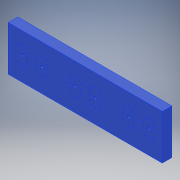
# Autodesk Inventor part: Gehaeuse_IN12_Fassung
Saved by Autodesk Inventor 2019 (Build 230136000, 136)
## iProperties
Created: 2019-10-07
Part Number: Gehaeuse_IN12_Fassung
Material: Generisch
Document SubType Name: Modeling
Designer: grubi
Density: 1 g/cm^3
Appearance: Vorgabe
Author: grubi
Autodesk Inventor part; units mm, degrees
ref_plane "YZ Plane" through (0, 0, 0) normal (1, 0, 0) x (0, 1, 0)
ref_plane "XZ Plane" through (0, 0, 0) normal (0, 1, 0) x (-1, 0, 0)
ref_plane "XY Plane" through (0, 0, 0) normal (0, 0, 1) x (1, 0, 0)
sketch "Skizze1" plane through (0, 0, 0) normal (0, 0, 1) x (1, 0, 0)
  spline S0 degree 3 poles (-66.4365, 60.4568) (-65.8605, 59.5154) (-65.2905, 58.8685) (-64.3775, 57.9498) (-63.6818, 57.3426) (-61.9226, 56.3485) (-61.068, 56.0155) (-59.0889, 55.5216) (-58.1394, 55.4718) (-57.6712, 55.4581) knots 0 0 0 0 0.331084 0.331084 0.698981 0.698981 1.004245 1.004245 1.384179 1.384179 1.384179 1.384179 projected
  line L0 (-57.6712, 55.4581) -> (-56.2137, 55.4552) projected
  spline S1 degree 3 poles (-56.2137, 55.4552) (-55.6042, 55.4706) (-54.6957, 55.5362) (-52.7979, 56.0044) (-51.9528, 56.3319) (-50.3662, 57.2202) (-49.6505, 57.7658) (-48.3993, 59.0179) (-47.8793, 59.6887) (-47.4285, 60.4187) knots 0 0 0 0 0.182919 0.182919 0.342589 0.342589 0.502166 0.502166 0.65206 0.65206 0.65206 0.65206 projected
  arc A0 (-47.4285, 60.4187) -> (-46.7276, 62.8786) centre (-51.4276, 62.888) ccw projected
  line L1 (-46.7276, 62.8786) -> (-46.6966, 78.3939) projected
  arc A1 (-46.6966, 78.3939) -> (-47.3876, 80.8565) centre (-51.3966, 78.4033) ccw projected
  spline S2 degree 3 poles (-47.3876, 80.8565) (-47.9637, 81.7979) (-48.5337, 82.4448) (-49.4467, 83.3635) (-50.1424, 83.9707) (-51.9015, 84.9648) (-52.7562, 85.2978) (-54.7353, 85.7917) (-55.6848, 85.8415) (-56.1529, 85.8552) knots 0 0 0 0 0.331084 0.331084 0.698981 0.698981 1.004245 1.004245 1.384179 1.384179 1.384179 1.384179 projected
  line L2 (-56.1529, 85.8552) -> (-57.6105, 85.8581) projected
  spline S3 degree 3 poles (-57.6105, 85.8581) (-58.22, 85.8427) (-59.1285, 85.7771) (-61.0263, 85.3089) (-61.8713, 84.9814) (-63.458, 84.0931) (-64.1737, 83.5475) (-65.4248, 82.2954) (-65.9449, 81.6246) (-66.3957, 80.8945) knots 0 0 0 0 0.182919 0.182919 0.342589 0.342589 0.502166 0.502166 0.65206 0.65206 0.65206 0.65206 projected
  arc A2 (-66.3957, 80.8945) -> (-67.0966, 78.4347) centre (-62.3966, 78.4253) ccw projected
  line L3 (-67.0966, 78.4347) -> (-67.1276, 62.9194) projected
  arc A3 (-67.1276, 62.9194) -> (-66.4365, 60.4568) centre (-62.4276, 62.91) ccw projected
  circle A4 centre (-60.9281, 62.6647) radius 0.5 projected
  circle A5 centre (-56.9301, 61.6567) radius 0.5 projected
  circle A6 centre (-52.9281, 62.6487) radius 0.5 projected
  circle A7 centre (-51.1711, 66.1452) radius 0.5 projected
  circle A8 centre (-51.1621, 70.6451) radius 0.5 projected
  circle A9 centre (-62.6711, 66.1682) radius 0.5 projected
  circle A10 centre (-62.6621, 70.6681) radius 0.5 projected
  circle A11 centre (-51.1531, 75.1451) radius 0.5 projected
  circle A12 centre (-52.8961, 78.6486) radius 0.5 projected
  circle A13 centre (-56.8941, 79.6566) radius 0.5 projected
  circle A14 centre (-62.6531, 75.1681) radius 0.5 projected
  circle A15 centre (-60.8961, 78.6646) radius 0.5 projected
  circle A16 centre (-56.9121, 70.6566) radius 1.45 projected
  spline S4 degree 3 poles (-45.6066, 60.4151) (-45.0305, 59.4738) (-44.4605, 58.8269) (-43.5475, 57.9082) (-42.8518, 57.3009) (-41.0927, 56.3068) (-40.2381, 55.9738) (-38.2589, 55.48) (-37.3094, 55.4301) (-36.8413, 55.4165) knots 0 0 0 0 0.331084 0.331084 0.698981 0.698981 1.004245 1.004245 1.384179 1.384179 1.384179 1.384179 projected
  line L4 (-36.8413, 55.4165) -> (-35.3838, 55.4136) projected
  spline S5 degree 3 poles (-35.3838, 55.4136) (-34.7742, 55.4289) (-33.8657, 55.4945) (-31.968, 55.9627) (-31.1229, 56.2903) (-29.5362, 57.1785) (-28.8206, 57.7241) (-27.5694, 58.9762) (-27.0493, 59.6471) (-26.5986, 60.3771) knots 0 0 0 0 0.182919 0.182919 0.342589 0.342589 0.502166 0.502166 0.65206 0.65206 0.65206 0.65206 projected
  arc A17 (-26.5986, 60.3771) -> (-25.8977, 62.8369) centre (-30.5977, 62.8463) ccw projected
  line L5 (-25.8977, 62.8369) -> (-25.8666, 78.3522) projected
  arc A18 (-25.8666, 78.3522) -> (-26.5577, 80.8149) centre (-30.5666, 78.3616) ccw projected
  spline S6 degree 3 poles (-26.5577, 80.8149) (-27.1337, 81.7562) (-27.7038, 82.4031) (-28.6167, 83.3218) (-29.3125, 83.929) (-31.0716, 84.9231) (-31.9262, 85.2561) (-33.9053, 85.75) (-34.8549, 85.7998) (-35.323, 85.8135) knots 0 0 0 0 0.331084 0.331084 0.698981 0.698981 1.004245 1.004245 1.384179 1.384179 1.384179 1.384179 projected
  line L6 (-35.323, 85.8135) -> (-36.7805, 85.8164) projected
  spline S7 degree 3 poles (-36.7805, 85.8164) (-37.39, 85.8011) (-38.2986, 85.7355) (-40.1963, 85.2672) (-41.0414, 84.9397) (-42.628, 84.0514) (-43.3437, 83.5058) (-44.5949, 82.2537) (-45.115, 81.5829) (-45.5657, 80.8529) knots 0 0 0 0 0.182919 0.182919 0.342589 0.342589 0.502166 0.502166 0.65206 0.65206 0.65206 0.65206 projected
  arc A19 (-45.5657, 80.8529) -> (-46.2666, 78.393) centre (-41.5666, 78.3836) ccw projected
  line L7 (-46.2666, 78.393) -> (-46.2976, 62.8777) projected
  arc A20 (-46.2976, 62.8777) -> (-45.6066, 60.4151) centre (-41.5976, 62.8683) ccw projected
  circle A21 centre (-40.0981, 62.623) radius 0.5 projected
  circle A22 centre (-36.1001, 61.615) radius 0.5 projected
  circle A23 centre (-32.0981, 62.607) radius 0.5 projected
  circle A24 centre (-30.3411, 66.1035) radius 0.5 projected
  circle A25 centre (-30.3321, 70.6035) radius 0.5 projected
  circle A26 centre (-41.8411, 66.1265) radius 0.5 projected
  circle A27 centre (-41.8321, 70.6265) radius 0.5 projected
  circle A28 centre (-30.3231, 75.1035) radius 0.5 projected
  circle A29 centre (-32.0661, 78.607) radius 0.5 projected
  circle A30 centre (-36.0641, 79.615) radius 0.5 projected
  circle A31 centre (-41.8231, 75.1265) radius 0.5 projected
  circle A32 centre (-40.0661, 78.623) radius 0.5 projected
  circle A33 centre (-36.0821, 70.615) radius 1.45 projected
  spline S8 degree 3 poles (-11.4366, 60.3468) (-10.8606, 59.4054) (-10.2906, 58.7585) (-9.3776, 57.8398) (-8.6819, 57.2326) (-6.9228, 56.2385) (-6.0681, 55.9055) (-4.089, 55.4116) (-3.1395, 55.3618) (-2.6714, 55.3481) knots 0 0 0 0 0.331084 0.331084 0.698981 0.698981 1.004245 1.004245 1.384179 1.384179 1.384179 1.384179 projected
  line L8 (-2.6714, 55.3481) -> (-1.2138, 55.3452) projected
  spline S9 degree 3 poles (-1.2138, 55.3452) (-0.6043, 55.3606) (0.3042, 55.4262) (2.202, 55.8944) (3.0471, 56.2219) (4.6337, 57.1102) (5.3494, 57.6558) (6.6006, 58.9079) (7.1206, 59.5787) (7.5714, 60.3088) knots 0 0 0 0 0.182919 0.182919 0.342589 0.342589 0.502166 0.502166 0.65206 0.65206 0.65206 0.65206 projected
  arc A34 (7.5714, 60.3088) -> (8.2723, 62.7686) centre (3.5723, 62.778) ccw projected
  line L9 (8.2723, 62.7686) -> (8.3033, 78.2839) projected
  arc A35 (8.3033, 78.2839) -> (7.6122, 80.7465) centre (3.6033, 78.2933) ccw projected
  spline S10 degree 3 poles (7.6122, 80.7465) (7.0362, 81.6879) (6.4662, 82.3348) (5.5532, 83.2535) (4.8575, 83.8607) (3.0984, 84.8548) (2.2437, 85.1878) (0.2646, 85.6817) (-0.6849, 85.7315) (-1.153, 85.7452) knots 0 0 0 0 0.331084 0.331084 0.698981 0.698981 1.004245 1.004245 1.384179 1.384179 1.384179 1.384179 projected
  line L10 (-1.153, 85.7452) -> (-2.6106, 85.7481) projected
  spline S11 degree 3 poles (-2.6106, 85.7481) (-3.2201, 85.7327) (-4.1286, 85.6671) (-6.0264, 85.1989) (-6.8715, 84.8714) (-8.4581, 83.9831) (-9.1738, 83.4375) (-10.425, 82.1854) (-10.945, 81.5146) (-11.3958, 80.7846) knots 0 0 0 0 0.182919 0.182919 0.342589 0.342589 0.502166 0.502166 0.65206 0.65206 0.65206 0.65206 projected
  arc A36 (-11.3958, 80.7846) -> (-12.0967, 78.3247) centre (-7.3967, 78.3153) ccw projected
  line L11 (-12.0967, 78.3247) -> (-12.1277, 62.8094) projected
  arc A37 (-12.1277, 62.8094) -> (-11.4366, 60.3468) centre (-7.4277, 62.8) ccw projected
  circle A38 centre (-5.9282, 62.5547) radius 0.5 projected
  circle A39 centre (-1.9302, 61.5467) radius 0.5 projected
  circle A40 centre (2.0718, 62.5387) radius 0.5 projected
  circle A41 centre (3.8288, 66.0352) radius 0.5 projected
  circle A42 centre (3.8378, 70.5352) radius 0.5 projected
  circle A43 centre (-7.6712, 66.0582) radius 0.5 projected
  circle A44 centre (-7.6622, 70.5582) radius 0.5 projected
  circle A45 centre (3.8468, 75.0351) radius 0.5 projected
  circle A46 centre (2.1038, 78.5386) radius 0.5 projected
  circle A47 centre (-1.8942, 79.5466) radius 0.5 projected
  circle A48 centre (-7.6532, 75.0581) radius 0.5 projected
  circle A49 centre (-5.8962, 78.5546) radius 0.5 projected
  circle A50 centre (-1.9122, 70.5467) radius 1.45 projected
  spline S12 degree 3 poles (9.3933, 60.3051) (9.9694, 59.3638) (10.5394, 58.7169) (11.4524, 57.7982) (12.1481, 57.1909) (13.9072, 56.1969) (14.7618, 55.8639) (16.7409, 55.37) (17.6905, 55.3202) (18.1586, 55.3065) knots 0 0 0 0 0.331084 0.331084 0.698981 0.698981 1.004245 1.004245 1.384179 1.384179 1.384179 1.384179 projected
  line L12 (18.1586, 55.3065) -> (19.6161, 55.3036) projected
  spline S13 degree 3 poles (19.6161, 55.3036) (20.2257, 55.3189) (21.1342, 55.3845) (23.0319, 55.8528) (23.877, 56.1803) (25.4636, 57.0685) (26.1793, 57.6142) (27.4305, 58.8662) (27.9506, 59.5371) (28.4013, 60.2671) knots 0 0 0 0 0.182919 0.182919 0.342589 0.342589 0.502166 0.502166 0.65206 0.65206 0.65206 0.65206 projected
  arc A51 (28.4013, 60.2671) -> (29.1022, 62.727) centre (24.4022, 62.7364) ccw projected
  line L13 (29.1022, 62.727) -> (29.1332, 78.2423) projected
  arc A52 (29.1332, 78.2423) -> (28.4422, 80.7049) centre (24.4333, 78.2517) ccw projected
  spline S14 degree 3 poles (28.4422, 80.7049) (27.8662, 81.6462) (27.2961, 82.2931) (26.3832, 83.2118) (25.6874, 83.8191) (23.9283, 84.8131) (23.0737, 85.1461) (21.0946, 85.64) (20.145, 85.6898) (19.6769, 85.7035) knots 0 0 0 0 0.331084 0.331084 0.698981 0.698981 1.004245 1.004245 1.384179 1.384179 1.384179 1.384179 projected
  line L14 (19.6769, 85.7035) -> (18.2194, 85.7064) projected
  spline S15 degree 3 poles (18.2194, 85.7064) (17.6099, 85.6911) (16.7013, 85.6255) (14.8036, 85.1573) (13.9585, 84.8297) (12.3719, 83.9415) (11.6562, 83.3958) (10.405, 82.1438) (9.8849, 81.4729) (9.4342, 80.7429) knots 0 0 0 0 0.182919 0.182919 0.342589 0.342589 0.502166 0.502166 0.65206 0.65206 0.65206 0.65206 projected
  arc A53 (9.4342, 80.7429) -> (8.7333, 78.2831) centre (13.4333, 78.2737) ccw projected
  line L15 (8.7333, 78.2831) -> (8.7023, 62.7677) projected
  arc A54 (8.7023, 62.7677) -> (9.3933, 60.3051) centre (13.4023, 62.7583) ccw projected
  circle A55 centre (14.9018, 62.513) radius 0.5 projected
  circle A56 centre (18.8998, 61.505) radius 0.5 projected
  circle A57 centre (22.9017, 62.497) radius 0.5 projected
  circle A58 centre (24.6587, 65.9935) radius 0.5 projected
  circle A59 centre (24.6677, 70.4935) radius 0.5 projected
  circle A60 centre (13.1588, 66.0165) radius 0.5 projected
  circle A61 centre (13.1678, 70.5165) radius 0.5 projected
  circle A62 centre (24.6767, 74.9935) radius 0.5 projected
  circle A63 centre (22.9337, 78.497) radius 0.5 projected
  circle A64 centre (18.9358, 79.505) radius 0.5 projected
  circle A65 centre (13.1768, 75.0165) radius 0.5 projected
  circle A66 centre (14.9338, 78.513) radius 0.5 projected
  circle A67 centre (18.9178, 70.505) radius 1.45 projected
  spline S16 degree 3 poles (43.5632, 60.2368) (44.1393, 59.2954) (44.7093, 58.6485) (45.6223, 57.7298) (46.318, 57.1226) (48.0771, 56.1285) (48.9318, 55.7955) (50.9109, 55.3016) (51.8604, 55.2518) (52.3285, 55.2382) knots 0 0 0 0 0.331084 0.331084 0.698981 0.698981 1.004245 1.004245 1.384179 1.384179 1.384179 1.384179 projected
  line L16 (52.3285, 55.2382) -> (53.786, 55.2352) projected
  spline S17 degree 3 poles (53.786, 55.2352) (54.3956, 55.2506) (55.3041, 55.3162) (57.2019, 55.7844) (58.0469, 56.1119) (59.6336, 57.0002) (60.3493, 57.5458) (61.6004, 58.7979) (62.1205, 59.4688) (62.5713, 60.1988) knots 0 0 0 0 0.182919 0.182919 0.342589 0.342589 0.502166 0.502166 0.65206 0.65206 0.65206 0.65206 projected
  arc A68 (62.5713, 60.1988) -> (63.2722, 62.6586) centre (58.5722, 62.668) ccw projected
  line L17 (63.2722, 62.6586) -> (63.3032, 78.1739) projected
  arc A69 (63.3032, 78.1739) -> (62.6121, 80.6366) centre (58.6032, 78.1833) ccw projected
  spline S18 degree 3 poles (62.6121, 80.6366) (62.0361, 81.5779) (61.4661, 82.2248) (60.5531, 83.1435) (59.8573, 83.7507) (58.0982, 84.7448) (57.2436, 85.0778) (55.2645, 85.5717) (54.3149, 85.6215) (53.8468, 85.6352) knots 0 0 0 0 0.331084 0.331084 0.698981 0.698981 1.004245 1.004245 1.384179 1.384179 1.384179 1.384179 projected
  line L18 (53.8468, 85.6352) -> (52.3893, 85.6381) projected
  spline S19 degree 3 poles (52.3893, 85.6381) (51.7798, 85.6227) (50.8713, 85.5571) (48.9735, 85.0889) (48.1284, 84.7614) (46.5418, 83.8731) (45.8261, 83.3275) (44.5749, 82.0754) (44.0549, 81.4046) (43.6041, 80.6746) knots 0 0 0 0 0.182919 0.182919 0.342589 0.342589 0.502166 0.502166 0.65206 0.65206 0.65206 0.65206 projected
  arc A70 (43.6041, 80.6746) -> (42.9032, 78.2147) centre (47.6032, 78.2053) ccw projected
  line L19 (42.9032, 78.2147) -> (42.8722, 62.6994) projected
  arc A71 (42.8722, 62.6994) -> (43.5632, 60.2368) centre (47.5722, 62.69) ccw projected
  circle A72 centre (49.0717, 62.4447) radius 0.5 projected
  circle A73 centre (53.0697, 61.4367) radius 0.5 projected
  circle A74 centre (57.0717, 62.4287) radius 0.5 projected
  circle A75 centre (58.8287, 65.9252) radius 0.5 projected
  circle A76 centre (58.8377, 70.4252) radius 0.5 projected
  circle A77 centre (47.3287, 65.9482) radius 0.5 projected
  circle A78 centre (47.3377, 70.4482) radius 0.5 projected
  circle A79 centre (58.8467, 74.9252) radius 0.5 projected
  circle A80 centre (57.1037, 78.4287) radius 0.5 projected
  circle A81 centre (53.1057, 79.4367) radius 0.5 projected
  circle A82 centre (47.3467, 74.9482) radius 0.5 projected
  circle A83 centre (49.1037, 78.4447) radius 0.5 projected
  circle A84 centre (53.0877, 70.4367) radius 1.45 projected
  spline S20 degree 3 poles (64.3932, 60.1951) (64.9692, 59.2538) (65.5393, 58.6069) (66.4522, 57.6882) (67.148, 57.081) (68.9071, 56.0869) (69.7617, 55.7539) (71.7408, 55.26) (72.6904, 55.2102) (73.1585, 55.1965) knots 0 0 0 0 0.331084 0.331084 0.698981 0.698981 1.004245 1.004245 1.384179 1.384179 1.384179 1.384179 projected
  line L20 (73.1585, 55.1965) -> (74.616, 55.1936) projected
  spline S21 degree 3 poles (74.616, 55.1936) (75.2255, 55.2089) (76.1341, 55.2745) (78.0318, 55.7428) (78.8769, 56.0703) (80.4635, 56.9586) (81.1792, 57.5042) (82.4304, 58.7563) (82.9505, 59.4271) (83.4012, 60.1571) knots 0 0 0 0 0.182919 0.182919 0.342589 0.342589 0.502166 0.502166 0.65206 0.65206 0.65206 0.65206 projected
  arc A85 (83.4012, 60.1571) -> (84.1021, 62.617) centre (79.4021, 62.6264) ccw projected
  line L21 (84.1021, 62.617) -> (84.1331, 78.1323) projected
  arc A86 (84.1331, 78.1323) -> (83.4421, 80.5949) centre (79.4331, 78.1417) ccw projected
  spline S22 degree 3 poles (83.4421, 80.5949) (82.866, 81.5362) (82.296, 82.1831) (81.383, 83.1018) (80.6873, 83.7091) (78.9282, 84.7032) (78.0736, 85.0362) (76.0945, 85.53) (75.1449, 85.5799) (74.6768, 85.5935) knots 0 0 0 0 0.331084 0.331084 0.698981 0.698981 1.004245 1.004245 1.384179 1.384179 1.384179 1.384179 projected
  line L22 (74.6768, 85.5935) -> (73.2193, 85.5964) projected
  spline S23 degree 3 poles (73.2193, 85.5964) (72.6097, 85.5811) (71.7012, 85.5155) (69.8035, 85.0473) (68.9584, 84.7197) (67.3718, 83.8315) (66.6561, 83.2859) (65.4049, 82.0338) (64.8848, 81.3629) (64.4341, 80.6329) knots 0 0 0 0 0.182919 0.182919 0.342589 0.342589 0.502166 0.502166 0.65206 0.65206 0.65206 0.65206 projected
  arc A87 (64.4341, 80.6329) -> (63.7332, 78.1731) centre (68.4332, 78.1637) ccw projected
  line L23 (63.7332, 78.1731) -> (63.7022, 62.6578) projected
  arc A88 (63.7022, 62.6578) -> (64.3932, 60.1951) centre (68.4021, 62.6484) ccw projected
  circle A89 centre (69.9017, 62.403) radius 0.5 projected
  circle A90 centre (73.8996, 61.395) radius 0.5 projected
  circle A91 centre (77.9016, 62.387) radius 0.5 projected
  circle A92 centre (79.6586, 65.8835) radius 0.5 projected
  circle A93 centre (79.6676, 70.3835) radius 0.5 projected
  circle A94 centre (68.1587, 65.9065) radius 0.5 projected
  circle A95 centre (68.1677, 70.4065) radius 0.5 projected
  circle A96 centre (79.6766, 74.8835) radius 0.5 projected
  circle A97 centre (77.9336, 78.387) radius 0.5 projected
  circle A98 centre (73.9356, 79.395) radius 0.5 projected
  circle A99 centre (68.1767, 74.9065) radius 0.5 projected
  circle A100 centre (69.9337, 78.403) radius 0.5 projected
  circle A101 centre (73.9176, 70.395) radius 1.45 projected
  line L24 (8.5956, 101.4703) -> (8.3793, 37.8364)
  line L25 (87.7471, 92.8448) -> (-70.7709, 92.8448)
  line L26 (-70.7709, 92.8448) -> (-70.7709, 46.8448)
  line L27 (-70.7709, 46.8448) -> (87.7471, 46.8448)
  line L28 (87.7471, 46.8448) -> (87.7471, 92.8448)
  line L29 (87.7471, 92.8448) -> (-70.7709, 46.8448) construction
  line L30 (-70.7709, 92.8448) -> (87.7471, 46.8448) construction
  line L31 (-12.3093, 46.9974) -> (32.6286, 46.9075) projected
  line L32 (32.8464, 92.2972) -> (-12.2185, 92.3873) projected
  point P0 (0, 0)
  point P1 (8.4881, 69.8448)
  dimension "d0" = 46
  constraints: 14 end point, 2 midpoint, 2 parallel, 1 horizontal, 1 perpendicular, 1 point on line, 3 other
  measures "d0" distance of L27.end L25.start
extrude "Extrusion2" add sketch "Skizze1" along normal blind 4 contours A3 L3 A2 S3 L2 S2 A1 L1 A0 S1 L0 S0 | A20 L7 A19 S7 L6 S6 A18 L5 A17 S5 L4 S4 | A37 L11 A36 S11 L10 S10 A35 L9 A34 S9 L8 S8 | A54 L15 A53 S15 L14 S14 A52 L13 A51 S13 L12 S12 | A71 L19 A70 S19 L18 S18 A69 L17 A68 S17 L16 S16 | A88 L23 A87 S23 L22 S22 A86 L21 A85 S21 L20 S20 | L25 L28 L27 L24 | L24 L27 L26 L25
sketch "Skizze2" plane through (0, 0, 4) normal (0, 0, 1) x (1, 0, 0)
  spline S0 degree 3 poles (73.1538, 54.8965) (72.9276, 54.903) (72.6988, 54.9155) (72.4727, 54.9339) (70.685, 55.0793) (68.9331, 55.6222) (67.4319, 56.598) (66.2444, 57.37) (65.2425, 58.3865) (64.4481, 59.5565) (64.3411, 59.7141) (64.2375, 59.8748) (64.1373, 60.0385) knots 0 0 0 0 0.000679 0.000679 0.000679 0.006047 0.006047 0.006047 0.010293 0.010293 0.010293 0.010865 0.010865 0.010865 0.010865 projected
  line L0 (74.6195, 54.8936) -> (73.1538, 54.8965) projected
  spline S1 degree 3 poles (83.6565, 59.9995) (83.5977, 59.9044) (83.5358, 59.807) (83.4115, 59.6178) (83.2216, 59.3372) (83.0208, 59.0664) (82.6043, 58.5384) (82.3068, 58.2044) (81.6695, 57.5748) (81.3297, 57.2792) (80.6038, 56.7301) (80.2221, 56.4801) (79.4273, 56.0341) (79.017, 55.8396) (78.1797, 55.5075) (77.7515, 55.3692) (76.877, 55.1452) (76.4287, 55.0593) (75.5277, 54.9393) (75.0747, 54.9049) (74.6195, 54.8936) knots 0 0 0 0 0.000335 0.000335 0.000671 0.001342 0.001342 0.002684 0.002684 0.004025 0.004025 0.005367 0.005367 0.006709 0.006709 0.008051 0.008051 0.009392 0.009392 0.010734 0.010734 0.010734 0.010734 projected
  arc A0 (83.6565, 59.9995) -> (84.4021, 62.6164) centre (79.4021, 62.6264) ccw projected
  line L1 (84.4331, 78.1317) -> (84.4021, 62.6164) projected
  arc A1 (84.4331, 78.1317) -> (83.698, 80.7515) centre (79.4331, 78.1417) ccw projected
  spline S2 degree 3 poles (74.6814, 85.8935) (74.9077, 85.887) (75.1365, 85.8746) (75.3626, 85.8562) (77.1503, 85.7107) (78.9022, 85.1678) (80.4033, 84.192) (81.5909, 83.42) (82.5928, 82.4036) (83.3872, 81.2336) (83.4942, 81.076) (83.5978, 80.9152) (83.698, 80.7515) knots 0 0 0 0 0.000679 0.000679 0.000679 0.006047 0.006047 0.006047 0.010293 0.010293 0.010293 0.010865 0.010865 0.010865 0.010865 projected
  line L2 (73.2158, 85.8964) -> (74.6814, 85.8935) projected
  spline S3 degree 3 poles (64.1788, 80.7905) (64.2376, 80.8857) (64.2995, 80.983) (64.4237, 81.1722) (64.6137, 81.4529) (64.8145, 81.7236) (65.231, 82.2516) (65.5285, 82.5856) (66.1658, 83.2152) (66.5056, 83.5108) (67.2315, 84.06) (67.6132, 84.3099) (68.4079, 84.7559) (68.8183, 84.9505) (69.6556, 85.2826) (70.0838, 85.4208) (70.9583, 85.6449) (71.4066, 85.7308) (72.3076, 85.8507) (72.7606, 85.8851) (73.2158, 85.8964) knots 0 0 0 0 0.000335 0.000335 0.000671 0.001342 0.001342 0.002684 0.002684 0.004025 0.004025 0.005367 0.005367 0.006709 0.006709 0.008051 0.008051 0.009392 0.009392 0.010734 0.010734 0.010734 0.010734 projected
  arc A2 (64.1788, 80.7905) -> (63.4332, 78.1737) centre (68.4332, 78.1637) ccw projected
  arc A3 (63.4022, 62.6584) -> (64.1373, 60.0385) centre (68.4021, 62.6484) ccw projected
  line L3 (63.4022, 62.6584) -> (63.4332, 78.1737) projected
  point P0 (0, 0)
extrude "Extrusion3" cut sketch "Skizze2" against normal through all
sketch "Skizze3" plane through (0, 0, 4) normal (0, 0, 1) x (1, 0, 0)
  spline S0 degree 3 poles (53.8515, 85.9352) (54.0777, 85.9287) (54.3065, 85.9162) (54.5327, 85.8978) (56.3203, 85.7524) (58.0723, 85.2095) (59.5734, 84.2336) (60.7609, 83.4616) (61.7628, 82.4452) (62.5572, 81.2752) (62.6642, 81.1176) (62.7678, 80.9569) (62.868, 80.7931) knots 0 0 0 0 0.000679 0.000679 0.000679 0.006047 0.006047 0.006047 0.010293 0.010293 0.010293 0.010865 0.010865 0.010865 0.010865 projected
  line L0 (52.3859, 85.9381) -> (53.8515, 85.9352) projected
  spline S1 degree 3 poles (43.3489, 80.8322) (43.4076, 80.9273) (43.4695, 81.0247) (43.5938, 81.2139) (43.7837, 81.4945) (43.9846, 81.7653) (44.4011, 82.2933) (44.6985, 82.6273) (45.3358, 83.2569) (45.6756, 83.5525) (46.4016, 84.1016) (46.7832, 84.3516) (47.578, 84.7976) (47.9883, 84.9921) (48.8256, 85.3242) (49.2538, 85.4625) (50.1283, 85.6865) (50.5766, 85.7724) (51.4776, 85.8924) (51.9306, 85.9268) (52.3859, 85.9381) knots 0 0 0 0 0.000335 0.000335 0.000671 0.001342 0.001342 0.002684 0.002684 0.004025 0.004025 0.005367 0.005367 0.006709 0.006709 0.008051 0.008051 0.009392 0.009392 0.010734 0.010734 0.010734 0.010734 projected
  arc A0 (43.3489, 80.8322) -> (42.6032, 78.2153) centre (47.6032, 78.2053) ccw projected
  line L1 (42.5722, 62.7) -> (42.6032, 78.2153) projected
  arc A1 (42.5722, 62.7) -> (43.3074, 60.0802) centre (47.5722, 62.69) ccw projected
  spline S2 degree 3 poles (52.3239, 54.9382) (52.0976, 54.9447) (51.8689, 54.9571) (51.6427, 54.9755) (49.8551, 55.121) (48.1031, 55.6639) (46.602, 56.6397) (45.4144, 57.4117) (44.4125, 58.4281) (43.6181, 59.5981) (43.5111, 59.7557) (43.4076, 59.9164) (43.3074, 60.0802) knots 0 0 0 0 0.000679 0.000679 0.000679 0.006047 0.006047 0.006047 0.010293 0.010293 0.010293 0.010865 0.010865 0.010865 0.010865 projected
  line L2 (53.7895, 54.9352) -> (52.3239, 54.9382) projected
  spline S3 degree 3 poles (62.8265, 60.0412) (62.7678, 59.946) (62.7058, 59.8487) (62.5816, 59.6594) (62.3916, 59.3788) (62.1908, 59.1081) (61.7743, 58.5801) (61.4769, 58.246) (60.8396, 57.6164) (60.4997, 57.3209) (59.7738, 56.7717) (59.3921, 56.5218) (58.5974, 56.0758) (58.1871, 55.8812) (57.3497, 55.5491) (56.9215, 55.4108) (56.0471, 55.1868) (55.5987, 55.1009) (54.6978, 54.981) (54.2448, 54.9465) (53.7895, 54.9352) knots 0 0 0 0 0.000335 0.000335 0.000671 0.001342 0.001342 0.002684 0.002684 0.004025 0.004025 0.005367 0.005367 0.006709 0.006709 0.008051 0.008051 0.009392 0.009392 0.010734 0.010734 0.010734 0.010734 projected
  arc A2 (62.8265, 60.0412) -> (63.5722, 62.658) centre (58.5722, 62.668) ccw projected
  line L3 (63.6032, 78.1733) -> (63.5722, 62.658) projected
  arc A3 (63.6032, 78.1733) -> (62.868, 80.7931) centre (58.6032, 78.1833) ccw projected
  point P0 (0, 0)
extrude "Extrusion4" cut sketch "Skizze3" against normal through all
sketch "Skizze4" plane through (0, 0, 4) normal (0, 0, 1) x (1, 0, 0)
  spline S0 degree 3 poles (19.6816, 86.0035) (19.9078, 85.997) (20.1366, 85.9846) (20.3627, 85.9662) (22.1504, 85.8207) (23.9023, 85.2778) (25.4035, 84.302) (26.591, 83.53) (27.5929, 82.5136) (28.3873, 81.3436) (28.4943, 81.1859) (28.5979, 81.0252) (28.6981, 80.8615) knots 0 0 0 0 0.000679 0.000679 0.000679 0.006047 0.006047 0.006047 0.010293 0.010293 0.010293 0.010865 0.010865 0.010865 0.010865 projected
  spline S1 degree 3 poles (18.2159, 86.0064) (18.21, 86.0063) (18.2038, 86.0061) (18.1971, 86.006) (18.1703, 86.0053) (18.1437, 86.0045) (18.1172, 86.0036) (18.0632, 86.0019) (18.0099, 85.9998) (17.9571, 85.9975) (17.8473, 85.9926) (17.7402, 85.9865) (17.6353, 85.9792) (17.4098, 85.9636) (17.1947, 85.9427) (16.985, 85.9171) (16.5342, 85.8619) (16.1111, 85.7864) (15.6701, 85.6799) (15.2325, 85.5742) (14.7906, 85.4387) (14.3636, 85.2757) (13.9278, 85.1095) (13.4975, 84.911) (13.0876, 84.6856) (12.2663, 84.2341) (11.5215, 83.6759) (10.8506, 83.0137) (10.2077, 82.3792) (9.6538, 81.6696) (9.1789, 80.9005) knots 0 0 0 0 0.000018 0.000018 0.000018 0.000088 0.000088 0.000088 0.000233 0.000233 0.000233 0.000534 0.000534 0.000534 0.001182 0.001182 0.001182 0.002574 0.002574 0.002574 0.003955 0.003955 0.003955 0.005365 0.005365 0.005365 0.008189 0.008189 0.008189 0.010895 0.010895 0.010895 0.010895 projected
  line L0 (18.2159, 86.0064) -> (19.6816, 86.0035) projected
  arc A0 (29.4332, 78.2417) -> (28.6981, 80.8615) centre (24.4333, 78.2517) ccw projected
  line L1 (29.4332, 78.2417) -> (29.4022, 62.7264) projected
  arc A1 (28.6566, 60.1095) -> (29.4022, 62.7264) centre (24.4022, 62.7364) ccw projected
  spline S2 degree 3 poles (28.6566, 60.1095) (28.5978, 60.0143) (28.5359, 59.917) (28.4117, 59.7278) (28.2217, 59.4472) (28.0209, 59.1764) (27.6044, 58.6484) (27.3069, 58.3144) (26.6696, 57.6848) (26.3298, 57.3892) (25.6039, 56.8401) (25.2222, 56.5901) (24.4275, 56.1441) (24.0171, 55.9496) (23.1798, 55.6174) (22.7516, 55.4792) (21.8771, 55.2552) (21.4288, 55.1692) (20.5278, 55.0493) (20.0748, 55.0149) (19.6196, 55.0036) knots 0 0 0 0 0.000335 0.000335 0.000671 0.001342 0.001342 0.002684 0.002684 0.004025 0.004025 0.005367 0.005367 0.006709 0.006709 0.008051 0.008051 0.009392 0.009392 0.010734 0.010734 0.010734 0.010734 projected
  line L2 (19.6196, 55.0036) -> (18.154, 55.0065) projected
  spline S3 degree 3 poles (18.154, 55.0065) (17.9277, 55.013) (17.6989, 55.0254) (17.4728, 55.0438) (15.6851, 55.1893) (13.9332, 55.7322) (12.4321, 56.708) (11.2445, 57.48) (10.2426, 58.4964) (9.4482, 59.6664) (9.3412, 59.8241) (9.2376, 59.9848) (9.1374, 60.1485) knots 0 0 0 0 0.000679 0.000679 0.000679 0.006047 0.006047 0.006047 0.010293 0.010293 0.010293 0.010865 0.010865 0.010865 0.010865 projected
  arc A2 (8.4023, 62.7683) -> (9.1374, 60.1485) centre (13.4023, 62.7583) ccw projected
  line L3 (8.4023, 62.7683) -> (8.4333, 78.2837) projected
  arc A3 (9.1789, 80.9005) -> (8.4333, 78.2837) centre (13.4333, 78.2737) ccw projected
  spline S4 degree 3 poles (-1.1484, 86.0452) (-0.9221, 86.0386) (-0.6934, 86.0262) (-0.4672, 86.0078) (1.3204, 85.8623) (3.0724, 85.3195) (4.5735, 84.3436) (5.761, 83.5716) (6.7629, 82.5552) (7.5573, 81.3852) (7.6644, 81.2276) (7.7679, 81.0669) (7.8681, 80.9031) knots 0 0 0 0 0.000679 0.000679 0.000679 0.006047 0.006047 0.006047 0.010293 0.010293 0.010293 0.010865 0.010865 0.010865 0.010865 projected
  line L4 (-2.614, 86.0481) -> (-1.1484, 86.0452) projected
  spline S5 degree 3 poles (-11.651, 80.9422) (-11.5923, 81.0373) (-11.5304, 81.1346) (-11.4061, 81.3239) (-11.2161, 81.6045) (-11.0153, 81.8752) (-10.5988, 82.4033) (-10.3014, 82.7373) (-9.6641, 83.3669) (-9.3242, 83.6625) (-8.5983, 84.2116) (-8.2166, 84.4615) (-7.4219, 84.9076) (-7.0116, 85.1021) (-6.1743, 85.4342) (-5.746, 85.5725) (-4.8716, 85.7965) (-4.4233, 85.8824) (-3.5223, 86.0024) (-3.0693, 86.0368) (-2.614, 86.0481) knots 0 0 0 0 0.000335 0.000335 0.000671 0.001342 0.001342 0.002684 0.002684 0.004025 0.004025 0.005367 0.005367 0.006709 0.006709 0.008051 0.008051 0.009392 0.009392 0.010734 0.010734 0.010734 0.010734 projected
  arc A4 (-11.651, 80.9422) -> (-12.3967, 78.3253) centre (-7.3967, 78.3153) ccw projected
  line L5 (-12.4277, 62.81) -> (-12.3967, 78.3253) projected
  arc A5 (-12.4277, 62.81) -> (-11.6925, 60.1902) centre (-7.4277, 62.8) ccw projected
  spline S6 degree 3 poles (-2.676, 55.0482) (-2.9023, 55.0547) (-3.131, 55.0671) (-3.3572, 55.0855) (-5.1448, 55.231) (-6.8968, 55.7739) (-8.3979, 56.7497) (-9.5854, 57.5217) (-10.5874, 58.5381) (-11.3817, 59.7081) (-11.4888, 59.8657) (-11.5923, 60.0264) (-11.6925, 60.1902) knots 0 0 0 0 0.000679 0.000679 0.000679 0.006047 0.006047 0.006047 0.010293 0.010293 0.010293 0.010865 0.010865 0.010865 0.010865 projected
  line L6 (-1.2104, 55.0452) -> (-2.676, 55.0482) projected
  spline S7 degree 3 poles (7.8266, 60.1511) (7.7679, 60.056) (7.7059, 59.9587) (7.5817, 59.7694) (7.3917, 59.4888) (7.1909, 59.2181) (6.7744, 58.6901) (6.477, 58.356) (5.8397, 57.7264) (5.4998, 57.4309) (4.7739, 56.8817) (4.3922, 56.6318) (3.5975, 56.1857) (3.1872, 55.9912) (2.3499, 55.6591) (1.9216, 55.5208) (1.0472, 55.2968) (0.5989, 55.2109) (-0.3021, 55.0909) (-0.7551, 55.0565) (-1.2104, 55.0452) knots 0 0 0 0 0.000335 0.000335 0.000671 0.001342 0.001342 0.002684 0.002684 0.004025 0.004025 0.005367 0.005367 0.006709 0.006709 0.008051 0.008051 0.009392 0.009392 0.010734 0.010734 0.010734 0.010734 projected
  arc A6 (7.8266, 60.1511) -> (8.5723, 62.768) centre (3.5723, 62.778) ccw projected
  line L7 (8.6033, 78.2833) -> (8.5723, 62.768) projected
  arc A7 (8.6033, 78.2833) -> (7.8681, 80.9031) centre (3.6033, 78.2933) ccw projected
  point P0 (0, 0)
extrude "Extrusion5" cut sketch "Skizze4" against normal through all contours A7 L7 A6 A2 L3 A3 | A3 L3 A2 A6 S7 L6 S6 A5 L5 A4 S5 L4 S4 A7
sketch "Skizze5" plane through (0, 0, 4) normal (0, 0, 1) x (1, 0, 0)
  spline S0 degree 3 poles (18.154, 55.0065) (17.9277, 55.013) (17.6989, 55.0254) (17.4728, 55.0438) (15.6851, 55.1893) (13.9332, 55.7322) (12.4321, 56.708) (11.2445, 57.48) (10.2426, 58.4964) (9.4482, 59.6664) (9.3412, 59.8241) (9.2376, 59.9848) (9.1374, 60.1485) knots 0 0 0 0 0.000679 0.000679 0.000679 0.006047 0.006047 0.006047 0.010293 0.010293 0.010293 0.010865 0.010865 0.010865 0.010865 projected
  line L0 (19.6196, 55.0036) -> (18.154, 55.0065) projected
  spline S1 degree 3 poles (28.6566, 60.1095) (28.5978, 60.0143) (28.5359, 59.917) (28.4117, 59.7278) (28.2217, 59.4472) (28.0209, 59.1764) (27.6044, 58.6484) (27.3069, 58.3144) (26.6696, 57.6848) (26.3298, 57.3892) (25.6039, 56.8401) (25.2222, 56.5901) (24.4275, 56.1441) (24.0171, 55.9496) (23.1798, 55.6174) (22.7516, 55.4792) (21.8771, 55.2552) (21.4288, 55.1692) (20.5278, 55.0493) (20.0748, 55.0149) (19.6196, 55.0036) knots 0 0 0 0 0.000335 0.000335 0.000671 0.001342 0.001342 0.002684 0.002684 0.004025 0.004025 0.005367 0.005367 0.006709 0.006709 0.008051 0.008051 0.009392 0.009392 0.010734 0.010734 0.010734 0.010734 projected
  arc A0 (28.6566, 60.1095) -> (29.4022, 62.7264) centre (24.4022, 62.7364) ccw projected
  line L1 (29.4332, 78.2417) -> (29.4022, 62.7264) projected
  arc A1 (29.4332, 78.2417) -> (28.6981, 80.8615) centre (24.4333, 78.2517) ccw projected
  spline S2 degree 3 poles (19.6816, 86.0035) (19.9078, 85.997) (20.1366, 85.9846) (20.3627, 85.9662) (22.1504, 85.8207) (23.9023, 85.2778) (25.4035, 84.302) (26.591, 83.53) (27.5929, 82.5136) (28.3873, 81.3436) (28.4943, 81.1859) (28.5979, 81.0252) (28.6981, 80.8615) knots 0 0 0 0 0.000679 0.000679 0.000679 0.006047 0.006047 0.006047 0.010293 0.010293 0.010293 0.010865 0.010865 0.010865 0.010865 projected
  spline S3 degree 3 poles (9.1789, 80.9005) (9.2377, 80.9957) (9.2996, 81.093) (9.4239, 81.2822) (9.6138, 81.5628) (9.8146, 81.8336) (10.2311, 82.3616) (10.5286, 82.6956) (11.1659, 83.3252) (11.5057, 83.6208) (12.2316, 84.1699) (12.6133, 84.4199) (13.4081, 84.8659) (13.8184, 85.0604) (14.6557, 85.3926) (15.0839, 85.5308) (15.9584, 85.7548) (16.4067, 85.8408) (17.3077, 85.9607) (17.7607, 85.9951) (18.2159, 86.0064) knots 0 0 0 0 0.000335 0.000335 0.000671 0.001342 0.001342 0.002684 0.002684 0.004025 0.004025 0.005367 0.005367 0.006709 0.006709 0.008051 0.008051 0.009392 0.009392 0.010734 0.010734 0.010734 0.010734 projected
  line L2 (18.2159, 86.0064) -> (19.6816, 86.0035) projected
  arc A2 (9.1789, 80.9005) -> (8.4333, 78.2837) centre (13.4333, 78.2737) ccw projected
  line L3 (8.4023, 62.7683) -> (8.4333, 78.2837) projected
  arc A3 (8.4023, 62.7683) -> (9.1374, 60.1485) centre (13.4023, 62.7583) ccw projected
  point P0 (0, 0)
extrude "Extrusion6" cut sketch "Skizze5" against normal through all
sketch "Skizze6" plane through (0, 0, 4) normal (0, 0, 1) x (1, 0, 0)
  line L0 (-35.3803, 55.1136) -> (-36.8459, 55.1165) projected
  spline S0 degree 3 poles (-26.3433, 60.2195) (-26.402, 60.1243) (-26.464, 60.027) (-26.5882, 59.8378) (-26.7782, 59.5571) (-26.979, 59.2864) (-27.3955, 58.7584) (-27.693, 58.4244) (-28.3303, 57.7948) (-28.6701, 57.4992) (-29.396, 56.95) (-29.7777, 56.7001) (-30.5724, 56.2541) (-30.9827, 56.0596) (-31.8201, 55.7274) (-32.2483, 55.5892) (-33.1228, 55.3651) (-33.5711, 55.2792) (-34.4721, 55.1593) (-34.9251, 55.1249) (-35.3803, 55.1136) knots 0 0 0 0 0.000335 0.000335 0.000671 0.001342 0.001342 0.002684 0.002684 0.004025 0.004025 0.005367 0.005367 0.006709 0.006709 0.008051 0.008051 0.009392 0.009392 0.010734 0.010734 0.010734 0.010734 projected
  arc A0 (-26.3433, 60.2195) -> (-25.5977, 62.8363) centre (-30.5977, 62.8463) ccw projected
  line L1 (-25.5666, 78.3516) -> (-25.5977, 62.8363) projected
  arc A1 (-25.5666, 78.3516) -> (-26.3018, 80.9715) centre (-30.5666, 78.3616) ccw projected
  spline S1 degree 3 poles (-35.3183, 86.1135) (-35.0921, 86.107) (-34.8633, 86.0946) (-34.6372, 86.0761) (-32.8495, 85.9307) (-31.0975, 85.3878) (-29.5964, 84.412) (-28.4089, 83.64) (-27.407, 82.6235) (-26.6126, 81.4535) (-26.5056, 81.2959) (-26.402, 81.1352) (-26.3018, 80.9715) knots 0 0 0 0 0.000679 0.000679 0.000679 0.006047 0.006047 0.006047 0.010293 0.010293 0.010293 0.010865 0.010865 0.010865 0.010865 projected
  line L2 (-36.7839, 86.1164) -> (-35.3183, 86.1135) projected
  spline S2 degree 3 poles (-45.821, 81.0105) (-45.7622, 81.1056) (-45.7003, 81.203) (-45.576, 81.3922) (-45.3861, 81.6728) (-45.1853, 81.9436) (-44.7688, 82.4716) (-44.4713, 82.8056) (-43.834, 83.4352) (-43.4942, 83.7308) (-42.7682, 84.2799) (-42.3866, 84.5299) (-41.5918, 84.9759) (-41.1815, 85.1704) (-40.3442, 85.5025) (-39.916, 85.6408) (-39.0415, 85.8648) (-38.5932, 85.9508) (-37.6922, 86.0707) (-37.2392, 86.1051) (-36.7839, 86.1164) knots 0 0 0 0 0.000335 0.000335 0.000671 0.001342 0.001342 0.002684 0.002684 0.004025 0.004025 0.005367 0.005367 0.006709 0.006709 0.008051 0.008051 0.009392 0.009392 0.010734 0.010734 0.010734 0.010734 projected
  arc A2 (-45.821, 81.0105) -> (-46.5666, 78.3936) centre (-41.5666, 78.3836) ccw projected
  line L3 (-46.5976, 62.8783) -> (-46.5666, 78.3936) projected
  arc A3 (-46.5976, 62.8783) -> (-45.8625, 60.2585) centre (-41.5976, 62.8683) ccw projected
  spline S3 degree 3 poles (-36.8459, 55.1165) (-37.0722, 55.123) (-37.301, 55.1354) (-37.5271, 55.1538) (-39.3147, 55.2993) (-41.0667, 55.8422) (-42.5678, 56.818) (-43.7554, 57.59) (-44.7573, 58.6064) (-45.5517, 59.7764) (-45.6587, 59.934) (-45.7623, 60.0948) (-45.8625, 60.2585) knots 0 0 0 0 0.000679 0.000679 0.000679 0.006047 0.006047 0.006047 0.010293 0.010293 0.010293 0.010865 0.010865 0.010865 0.010865 projected
  point P0 (0, 0)
extrude "Extrusion7" cut sketch "Skizze6" against normal through all
sketch "Skizze7" plane through (0, 0, 4) normal (0, 0, 1) x (1, 0, 0)
  spline S0 degree 3 poles (-47.1733, 60.2611) (-47.232, 60.166) (-47.2939, 60.0687) (-47.4182, 59.8794) (-47.6081, 59.5988) (-47.809, 59.3281) (-48.2255, 58.8) (-48.5229, 58.466) (-49.1602, 57.8364) (-49.5001, 57.5408) (-50.226, 56.9917) (-50.6077, 56.7418) (-51.4024, 56.2957) (-51.8127, 56.1012) (-52.65, 55.7691) (-53.0782, 55.6308) (-53.9527, 55.4068) (-54.401, 55.3209) (-55.302, 55.2009) (-55.755, 55.1665) (-56.2103, 55.1552) knots 0 0 0 0 0.000335 0.000335 0.000671 0.001342 0.001342 0.002684 0.002684 0.004025 0.004025 0.005367 0.005367 0.006709 0.006709 0.008051 0.008051 0.009392 0.009392 0.010734 0.010734 0.010734 0.010734 projected
  line L0 (-56.2103, 55.1552) -> (-57.6759, 55.1581) projected
  spline S1 degree 3 poles (-57.6759, 55.1581) (-57.9022, 55.1647) (-58.1309, 55.1771) (-58.3571, 55.1955) (-60.1447, 55.341) (-61.8967, 55.8838) (-63.3978, 56.8597) (-64.5853, 57.6317) (-65.5872, 58.6481) (-66.3816, 59.8181) (-66.4886, 59.9757) (-66.5922, 60.1364) (-66.6924, 60.3002) knots 0 0 0 0 0.000679 0.000679 0.000679 0.006047 0.006047 0.006047 0.010293 0.010293 0.010293 0.010865 0.010865 0.010865 0.010865 projected
  arc A0 (-67.4276, 62.92) -> (-66.6924, 60.3002) centre (-62.4276, 62.91) ccw projected
  line L1 (-67.4276, 62.92) -> (-67.3966, 78.4353) projected
  arc A1 (-66.6509, 81.0522) -> (-67.3966, 78.4353) centre (-62.3966, 78.4253) ccw projected
  spline S2 degree 3 poles (-66.6509, 81.0522) (-66.5922, 81.1473) (-66.5302, 81.2446) (-66.406, 81.4339) (-66.216, 81.7145) (-66.0152, 81.9852) (-65.5987, 82.5132) (-65.3013, 82.8473) (-64.664, 83.4769) (-64.3241, 83.7724) (-63.5982, 84.3216) (-63.2165, 84.5715) (-62.4218, 85.0176) (-62.0115, 85.2121) (-61.1742, 85.5442) (-60.7459, 85.6825) (-59.8715, 85.9065) (-59.4232, 85.9924) (-58.5222, 86.1124) (-58.0692, 86.1468) (-57.6139, 86.1581) knots 0 0 0 0 0.000335 0.000335 0.000671 0.001342 0.001342 0.002684 0.002684 0.004025 0.004025 0.005367 0.005367 0.006709 0.006709 0.008051 0.008051 0.009392 0.009392 0.010734 0.010734 0.010734 0.010734 projected
  line L2 (-57.6139, 86.1581) -> (-56.1483, 86.1551) projected
  spline S3 degree 3 poles (-56.1483, 86.1551) (-55.922, 86.1486) (-55.6933, 86.1362) (-55.4671, 86.1178) (-53.6795, 85.9723) (-51.9275, 85.4294) (-50.4264, 84.4536) (-49.2388, 83.6816) (-48.2369, 82.6652) (-47.4426, 81.4952) (-47.3355, 81.3376) (-47.232, 81.1769) (-47.1318, 81.0131) knots 0 0 0 0 0.000679 0.000679 0.000679 0.006047 0.006047 0.006047 0.010293 0.010293 0.010293 0.010865 0.010865 0.010865 0.010865 projected
  arc A2 (-46.3966, 78.3933) -> (-47.1318, 81.0131) centre (-51.3966, 78.4033) ccw projected
  line L3 (-46.3966, 78.3933) -> (-46.4276, 62.878) projected
  arc A3 (-47.1733, 60.2611) -> (-46.4276, 62.878) centre (-51.4276, 62.888) ccw projected
  point P0 (0, 0)
extrude "Extrusion8" cut sketch "Skizze7" against normal through all
